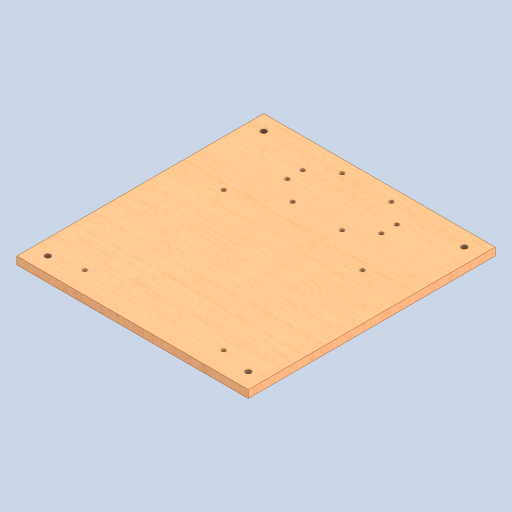
# Autodesk Inventor part: Base madeira
Saved by Autodesk Inventor 2023 (Build 270158000, 158)
## iProperties
Created: 2023-04-12
Part Number: Base madeira
Material: Wood (Cherry)
Document SubType Name: Sheet Metal
Designer: Mateus PC
Density: 0.63 g/cm^3
Sheet Metal Rule: Default_mm
Appearance: Cerejeira - Natural com pouco brilho
Mass: 602.308 g
Surface Area: 2063.9 cm^2
Volume: 956.045 cm^3
Author: Mateus PC
Autodesk Inventor part; units mm, degrees
ref_plane "YZ Plane" through (0, 0, 0) normal (1, 0, 0) x (0, 1, 0)
ref_plane "XZ Plane" through (0, 0, 0) normal (0, 1, 0) x (-1, 0, 0)
ref_plane "XY Plane" through (0, 0, 0) normal (0, 0, 1) x (1, 0, 0)
sketch "Esboço1" plane through (0, 0, 0) normal (0, 1, 0) x (-1, 0, 0)
  line L0 (0, 0) -> (300, 0)
  line L1 (300, 0) -> (300, -320)
  line L2 (300, -320) -> (0, -320)
  line L3 (0, -320) -> (0, 0)
  dimension "d0" = 300
  dimension "d1" = 320
  constraints: 8 end point, 2 parallel, 1 horizontal, 1 perpendicular
  measures "d0" distance of L1.end L2.end
  measures "d1" distance of L0.end L1.end
extrude "Extrusão1" add sketch "Esboço1" along normal blind 10
sketch "Sketch2" plane through (0, 10, 0) normal (0, 1, 0) x (1, 0, 0)
  line L0 (-300, 320) -> (-300, 0)
  line L1 (-300, 0) -> (0, 0)
  line L2 (0, 320) -> (-300, 320)
  line L3 (0, 0) -> (0, 320)
  point P0 (-182, 239.6)
  point P1 (-182, 303.6)
  point P2 (-118, 239.6)
  point P3 (-118, 303.6)
  point P4 (-211, 281.6)
  point P5 (-89, 281.6)
  point P6 (-211, 261.6)
  point P7 (-89, 261.6)
  point P8 (-240, 28.1)
  point P9 (-240, 208.1)
  point P10 (-60, 28.1)
  point P11 (-60, 208.1)
  dimension "d16" = 64
  dimension "d17" = 64
  dimension "d18" = 300
  dimension "d19" = 320
  dimension "d20" = 16.4
  dimension "d21" = 118
  dimension "d22" = 122
  dimension "d23" = 20
  dimension "d24" = 38.4
  dimension "d25" = 89
  dimension "d26" = 180
  dimension "d27" = 180
  dimension "d28" = 60
  dimension "d29" = 28.1
  constraints: 8 end point, 3 horizontal, 3 vertical, 9 other
  measures "d16" distance of point (-182, 239.6) point (-182, 303.6)
  measures "d17" distance of point (-182, 239.6) point (-118, 239.6)
  measures "d18" distance of L0.end L1.end
  measures "d19" distance of L0.start L0.end
  measures "d20" distance from line of L2 point (-182, 303.6)
  measures "d21" distance from line of L3 point (-118, 303.6)
  measures "d22" distance of point (-211, 281.6) point (-89, 281.6)
  measures "d23" distance of point (-211, 281.6) point (-211, 261.6)
  measures "d24" distance from line of L2 point (-211, 281.6)
  measures "d25" distance from line of L0 point (-211, 261.6)
  measures "d26" distance of point (-240, 28.1) point (-240, 208.1)
  measures "d27" distance of point (-240, 28.1) point (-60, 28.1)
  measures "d28" distance from line of L0 point (-240, 28.1)
  measures "d29" distance from line of L1 point (-240, 28.1)
hole "Hole1" at (-60, 10, -208.1) at (-60, 10, -28.1) at (-240, 10, -208.1) at (-240, 10, -28.1) at (-89, 10, -261.6) at (-211, 10, -261.6) at (-89, 10, -281.6) at (-211, 10, -281.6) at (-118, 10, -303.6) at (-118, 10, -239.6) at (-182, 10, -303.6) at (-182, 10, -239.6) direction (0, -1, 0) diameter 5 end through all
sketch "Sketch3" plane through (0, 10, 0) normal (0, 1, 0) x (1, 0, 0)
  line L0 (-300, 320) -> (-300, 0)
  line L1 (-300, 0) -> (0, 0)
  point P0 (-280, 20)
  point P1 (-280, 300)
  point P2 (-20, 20)
  point P3 (-20, 300)
  dimension "d41" = 280
  dimension "d42" = 260
  dimension "d43" = 320
  dimension "d44" = 300
  dimension "d45" = 20
  dimension "d46" = 20
  constraints: 4 end point, 1 horizontal, 1 vertical, 3 other
  measures "d41" distance of point (-280, 20) point (-280, 300)
  measures "d42" distance of point (-280, 20) point (-20, 20)
  measures "d43" distance of L0.start L0.end
  measures "d44" distance of L0.end L1.end
  measures "d45" distance from line of L1 point (-280, 20)
  measures "d46" distance from line of L0 point (-280, 20)
hole "Hole2" at (-20, 10, -300) at (-20, 10, -20) at (-280, 10, -300) at (-280, 10, -20) direction (0, -1, 0) diameter 7.134 end through all thread size "M8x0.8" class "6H" standard "ISO Metric profile"
equation "\"d21\" = -0.5 * d17 + 0.5 * d18"
equation "\"d25\" = 0.5 * d18 - 0.5 * d22"
equation "\"d28\" = 0.5 * d18 - 0.5 * d27"
equation "\"d35\" = Espessura"
equation "\"d45\" = 0.5 * d43 - 0.5 * d41"
equation "\"d46\" = 0.5 * d44 - 0.5 * d42"
equation "\"Raio_vergadura\" = Espessura"
equation "\"Largura_alívio_de_vergadura\" = Espessura"
equation "\"Profundidade_alívio_de_vergadura\" = 0.5 * Espessura"
equation "\"Tamanho_alívio_de_dobra\" = 4 * Espessura"
equation "\"Remanescente_mínimo\" = 2 * Espessura"
equation "\"Raiodetransição\" = Raio_vergadura"
equation "\"Tamanho_de_raio_de_Jacobi\" = Raio_vergadura"
equation "\"TamanhoFolga\" = Espessura"
equation "\"Espessura\" = 0.5"
